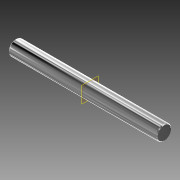
# Autodesk Inventor part: D-034
Saved by Autodesk Inventor 2015 (Build 190159000, 159)
## iProperties
Company: MARCHA TECHNOLOGY
Created: 2013-10-24
Part Number: D-034
Document SubType Name: Modeling
Designer: O.Martin
Density: 7.85 g/cm^3
Project: WITBOXprinter_K01
Stock Number: 28655
Material: Steel
Description: BARRA  DELANTERA
Mass: 7.69927 g
Surface Area: 8.19905 cm^2
Volume: 0.980799 cm^3
Appearance: Chrome - Polished Black
Author: O.Martin
Autodesk Inventor part; units mm, degrees
ref_plane "XZ Plane" through (0, 0, 0) normal (0, 1, 0) x (-1, 0, 0)
ref_plane "XY Plane" through (0, 0, 0) normal (0, 0, 1) x (1, 0, 0)
sketch "Boceto1" plane through (0, 0, 0) normal (0, 0, 1) x (1, 0, 0)
  line L0 (-25, 2.5) -> (25, 2.5)
  line L1 (25, 2.5) -> (25, 0)
  line L2 (25, 0) -> (-25, 0)
  line L3 (-25, 0) -> (-25, 2.5)
  point P0 (0, 0)
  point P1 (0, 0)
  dimension "d0" = 5
  dimension "d1" = 50
  constraints: 8 end point, 2 parallel, 1 coincident, 1 horizontal, 1 midpoint, 1 perpendicular
  measures "d0" diameter of L0 L2
  measures "d1" distance of L1.end L2.end
revolve "Revolución1" add sketch "Boceto1" angle 360 about axis through (25, 0, 0) along (-1, 0, 0)
chamfer "Chaflán1" distance 0.25 angle 45 2 edges at (-25, -2.5, 0) (25, -2.5, 0)
body "Solid1"
